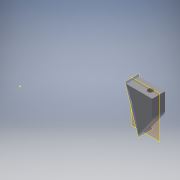
# Autodesk Inventor part: light_mount
Saved by Autodesk Inventor 2016 (Build 200138000, 138)
## iProperties
Created: 2017-09-25
Part Number: light_mount
Material: Generic
Document SubType Name: Modeling
Designer: Student
Density: 1 g/cm^3
Appearance: Default
Author: Student
Autodesk Inventor part; units mm, degrees
ref_plane "YZ Plane" through (0, 0, 0) normal (1, 0, 0) x (0, 1, 0)
ref_plane "XZ Plane" through (0, 0, 0) normal (0, 1, 0) x (-1, 0, 0)
ref_plane "XY Plane" through (0, 0, 0) normal (0, 0, 1) x (1, 0, 0)
sketch "Sketch1" plane through (0, 0, 0) normal (0, 0, 1) x (1, 0, 0)
  arc A0 (184.5073, 35.0953) -> (33.1465, 192.9611) centre (-3.7688, 6.072) ccw construction
  arc A1 (184.5073, 35.0953) -> (166.6077, 91.29) centre (-3.7688, 6.072) ccw
  line L0 (202.6605, 59.7837) -> (184.5073, 35.0953)
  arc A2 (202.6605, 59.7837) -> (205.1287, 67.3071) centre (192.4287, 67.3071) ccw
  line L1 (166.6077, 91.29) -> (205.1287, 91.29)
  line L2 (205.1287, 67.3071) -> (205.1287, 91.29)
  point P0 (0, 0)
  dimension "d3" = 12.7
  constraints: 7 point on circle, 6 end point, 3 centre point, 1 concentric, 1 horizontal, 1 perpendicular, 1 tangent, 1 other
  measures "d3" radius of A2
extrude "Extrusion1" add sketch "Sketch1" along normal mid plane 19.05
sketch "Sketch2" plane through (166.6077, 91.29, 9.525) normal (0, 1, 0) x (1, 0, 0)
  circle A0 centre (26.5011, 9.525) radius 3.81
  line L0 (38.5211, 0) -> (38.5211, 19.05) construction
  ellipse E0 centre (26.5011, 5.9613) end of major axis (22.6972, 5.7462) minor radius 3.81 construction
  ellipse E1 centre (26.5011, 5.9613) end of major axis (22.6972, 5.7462) minor radius 3.81 construction
  point P0 (-166.6077, 9.525)
  point P1 (38.5211, 9.525)
  dimension "d6" = 7.62
  constraints: 1 centre point, 1 horizontal alignment, 1 midpoint, 1 vertical alignment, 2 other
  measures "d6" diameter of A0
extrude "Extrusion2" cut sketch "Sketch2" against normal blind 25.4
ref_plane "Work Plane1" through (166.6077, 91.29, 9.525) normal (-0.9528, -0.3035, 0) x (0, 0, -1)
sketch "Sketch3" plane through (166.6077, 91.29, 9.525) normal (-0.9528, -0.3035, 0) x (0, 0, -1)
  circle A0 centre (9.525, 12.7) radius 2.921
  line L0 (0, 0) -> (19.05, 0) construction
  circle A1 centre (9.525, 38.6566) radius 2.921
  line L1 (19.05, 58.9766) -> (0, 58.9766) projected
  point P0 (9.525, 36.4178)
  point P1 (9.525, 0)
  point P2 (9.525, 0)
  dimension "d9" = 5.842
  dimension "d10" = 12.7
  dimension "d11" = 5.842
  dimension "d12" = 20.32
  constraints: 2 centre point, 2 midpoint, 2 vertical alignment
  measures "d9" diameter of A0
  measures "d10" distance from line of L0 A0.centre
  measures "d11" diameter of A1
  measures "d12" distance from line of A1.centre L1
extrude "Extrusion3" cut sketch "Sketch3" against normal blind 10.16
ref_plane "Work Plane2" through (0, 0, 0) normal (0, 0, 1) x (1, 0, 0)
sketch "Sketch4" plane through (0, 0, 0) normal (0, 0, 1) x (1, 0, 0)
  point P0 (0, 0)
equation "\"d11\" = d9"
body "Solid1"
